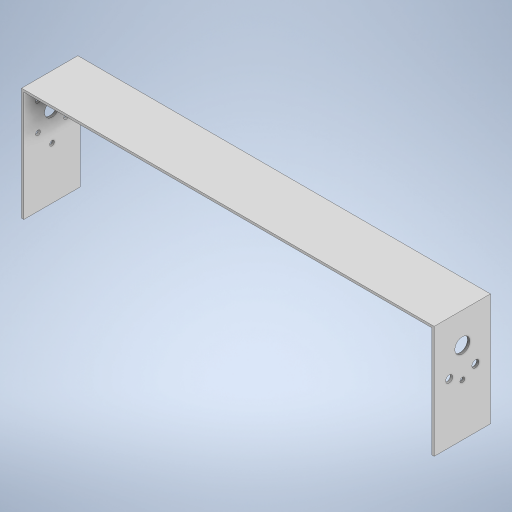
# Autodesk Inventor part: Bracket
Saved by Autodesk Inventor 2024 (Build 280153000, 153)
## iProperties
Created: 2025-01-21
Part Number: Bracket
Material: Generic
Document SubType Name: Modeling
Designer: Sven
Density: 1 g/cm^3
Appearance: Default
Author: Sven
Autodesk Inventor part; units mm, degrees
ref_plane "YZ Plane" through (0, 0, 0) normal (1, 0, 0) x (0, 1, 0)
ref_plane "XZ Plane" through (0, 0, 0) normal (0, 1, 0) x (-1, 0, 0)
ref_plane "XY Plane" through (0, 0, 0) normal (0, 0, 1) x (1, 0, 0)
sketch "Sketch1" plane through (0, 0, 0) normal (0, 0, 1) x (1, 0, 0)
  line L0 (-139.7, 38.1) -> (139.7, 38.1)
  line L1 (139.7, 38.1) -> (139.7, -38.1)
  line L2 (139.7, -38.1) -> (-139.7, -38.1)
  line L3 (-139.7, -38.1) -> (-139.7, 38.1)
  point P0 (0, 0)
  point P1 (0, 38.1)
  point P2 (139.7, 0)
  dimension "d0" = 279.4
  dimension "d1" = 76.2
  constraints: 8 end point, 2 midpoint, 2 parallel, 1 horizontal, 1 horizontal alignment, 1 perpendicular, 1 vertical alignment
  measures "d0" distance of L0.start L0.end
  measures "d1" distance of L0.end L1.end
extrude "Extrusion1" add sketch "Sketch1" along normal blind 38.1
sketch "Sketch2" plane through (0, 0, 38.1) normal (0, 0, 1) x (1, 0, 0)
  line L0 (-139.7, -38.1) -> (139.7, -38.1) projected
  line L1 (-138.1125, 36.5125) -> (138.1125, 36.5125)
  line L2 (138.1125, 36.5125) -> (138.1125, -38.1)
  line L3 (138.1125, -38.1) -> (-138.1125, -38.1)
  line L4 (-138.1125, -38.1) -> (-138.1125, 36.5125)
  line L5 (139.7, -38.1) -> (139.7, 38.1) projected
  line L6 (139.7, 38.1) -> (-139.7, 38.1) projected
  line L7 (-139.7, 38.1) -> (-139.7, -38.1) projected
  point P0 (0, 0)
  point P1 (-138.1125, -38.1)
  dimension "d4" = 1.5875
  dimension "d5" = 1.5875
  dimension "d6" = 1.5875
  constraints: 8 end point, 2 parallel, 1 horizontal, 1 perpendicular, 1 point on line
  measures "d4" distance between parallel lines of L5 L2
  measures "d5" distance between parallel lines of L6 L1
  measures "d6" distance between parallel lines of L7 L4
extrude "Extrusion2" cut sketch "Sketch2" against normal up to surface (38.1 mm away) contours L4 L1 L2 L0
sketch "Sketch3" plane through (-138.1125, -38.1, 38.1) normal (1, 0, 0) x (0, 0, -1)
  circle A0 centre (19.05, 55.5625) radius 5.05
  line L0 (0, 74.6125) -> (38.1, 74.6125) projected
  circle A1 centre (19.05, 35.2425) radius 1.5875
  line L1 (38.1, 76.2) -> (0, 76.2) projected
  point P0 (38.1, 38.1)
  point P1 (19.05, 76.2)
  dimension "d9" = 10.1
  dimension "d10" = 19.05
  dimension "d13" = 3.175
  dimension "d15" = 20.32
  constraints: 2 centre point, 2 vertical alignment, 1 midpoint
  measures "d9" diameter of A0
  measures "d10" distance from line of L0 A0.centre
  measures "d13" diameter of A1
  measures "d15" distance of A1.centre A0.centre
extrude "Extrusion3" cut sketch "Sketch3" along normal through all both and the other way through all
sketch "Sketch4" plane through (139.7, -38.1, 0) normal (1, 0, 0) x (0, 0, -1)
  circle A0 centre (-10.16, 40.3225) radius 2.3813
  line L0 (0, 76.2) -> (-38.1, 76.2) construction
  line L1 (-19.05, 76.2) -> (-19.05, -3.1611) construction
  line L2 (0, 0) -> (0, 76.2) projected
  circle A1 centre (-19.05, 55.5625) radius 5.05 projected
  circle A2 centre (-27.94, 40.3225) radius 2.3813
  point P0 (0, 38.1)
  dimension "d16" = 10.16
  dimension "d17" = 15.24
  dimension "d18" = 4.7625
  constraints: 2 centre point, 2 end point, 1 midpoint, 1 symmetric about line, 1 vertical, 1 other
  measures "d16" distance from line of L2 A0.centre
  measures "d17" vertical distance of A1.centre A0.centre
  measures "d18" diameter of A0
extrude "Extrusion4" cut sketch "Sketch4" against normal up to surface (1.5875 mm away) contours A0 | A2
sketch "Sketch5" plane through (-139.7, -38.1, 0) normal (-1, 0, 0) x (0, 0, 1)
  circle A0 centre (19.05, 55.5625) radius 5.05 construction
  line L0 (19.05, 55.5625) -> (19.05, 80.4525) construction
  line L1 (19.05, 55.5625) -> (48.6825, 55.5625) construction
  circle A1 centre (28.575, 65.0875) radius 1.5875
  circle A2 centre (9.525, 65.0875) radius 1.5875
  circle A3 centre (28.575, 46.0375) radius 1.5875
  circle A4 centre (9.525, 46.0375) radius 1.5875
  point P0 (0, 38.1)
  dimension "d21" = 3.175
  dimension "d22" = 9.525
  dimension "d23" = 9.525
  constraints: 4 centre point, 4 end point, 3 symmetric about line, 1 horizontal, 1 vertical, 3 other
  measures "d21" diameter of A1
  measures "d22" distance from line of L1 A1.centre
  measures "d23" distance from line of L0 A1.centre
extrude "Extrusion5" cut sketch "Sketch5" against normal up to surface (1.5875 mm away)
body "Solid1"
